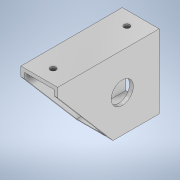
# Autodesk Inventor part: SU22_SQP_20_40_EU_sn
Saved by Autodesk Inventor 2022 (Build 260153000, 153)
## iProperties
Created: 2022-06-28
Part Number: SU22_SQP_20_40_EU_sn
Material: アルミニウム 6061-AHC
Document SubType Name: Modeling
Designer: 中島 青蔵
Density: 2.7 g/cm^3
Appearance: アルミニウム - ダーク
Author: 中島 青蔵
Autodesk Inventor part; units mm, degrees
ref_plane "YZ Plane" through (0, 0, 0) normal (1, 0, 0) x (0, 1, 0)
ref_plane "XZ Plane" through (0, 0, 0) normal (0, 1, 0) x (-1, 0, 0)
ref_plane "XY Plane" through (0, 0, 0) normal (0, 0, 1) x (1, 0, 0)
sketch "スケッチ1" plane through (0, 0, 0) normal (0, 0, 1) x (1, 0, 0)
  line L0 (0, 0) -> (20, 0)
  line L1 (20, 0) -> (20, 40)
  line L2 (20, 40) -> (0, 40)
  line L3 (0, 40) -> (0, 0)
  line L4 (2, 2) -> (18, 2)
  line L5 (18, 2) -> (18, 38)
  line L6 (18, 38) -> (2, 38)
  line L7 (2, 38) -> (2, 2)
  dimension "d0" = 20
  dimension "d1" = 40
  dimension "d2" = 2
  constraints: 16 end point, 3 other
  measures "d0" distance of L2.end L1.end
  measures "d1" distance of L1.end L0.end
  measures "d2" distance between parallel lines of L3 L7
extrude "押し出し1" add sketch "スケッチ1" along normal blind 55
sketch "スケッチ2" plane through (20, 0, 0) normal (1, 0, 0) x (0, 0, -1)
  line L0 (0, 0) -> (0, 40) projected
  point P0 (-20, 20)
  dimension "d5" = 20
  measures "d5" distance from line of L0 point (-20, 20)
hole "穴1" at (20, 20, 20) direction (-1, 0, 0) diameter 12 depth 2
sketch "スケッチ3" plane through (0, 0, 0) normal (-1, 0, 0) x (0, 0, 1)
  line L0 (0, 40) -> (0, 0) projected
  line L1 (0, 40) -> (55, 40) projected
  point P0 (20, 20)
  point P1 (20, 11)
  point P2 (20, 29)
  dimension "d13" = 20
  dimension "d14" = 20
  dimension "d15" = 9
  dimension "d16" = 9
  constraints: 2 vertical alignment
  measures "d13" distance from line of L0 point (20, 20)
  measures "d14" distance from line of L1 point (20, 20)
  measures "d15" distance of point (20, 20) point (20, 11)
  measures "d16" distance of point (20, 20) point (20, 29)
hole "穴2" at (0, 20, 20) direction (1, 0, 0) diameter 12 depth 2
hole "穴3" at (0, 11, 20) at (0, 29, 20) direction (1, 0, 0) diameter 3.1 depth 2
sketch "スケッチ4" plane through (0, 40, 0) normal (0, 1, 0) x (1, 0, 0)
  line L0 (20, 0) -> (0, 0) projected
  point P0 (10, -7.5)
  point P1 (10, -47.5)
  dimension "d31" = 7.5
  dimension "d32" = 47.5
  measures "d31" distance from line of L0 point (10, -7.5)
  measures "d32" distance from line of L0 point (10, -47.5)
hole "穴4" at (10, 40, 7.5) at (10, 40, 47.5) direction (0, -1, 0) diameter 3.1 depth 2
sketch "スケッチ5" plane through (0, 0, 0) normal (-1, 0, 0) x (0, 0, 1)
  line L0 (0, 0) -> (55, 0) projected
  line L1 (25, 0) -> (55, 35)
  line L2 (55, 2) -> (55, 38) projected
  line L3 (55, 40) -> (55, 0) projected
  dimension "d40" = 30
  dimension "d41" = 35
  constraints: 2 end point, 2 point on line
  measures "d40" distance from line of L3 L1.start
  measures "d41" distance from line of L0 L1.end
extrude "押し出し2" cut sketch "スケッチ5" against normal blind 55
equation "\"d16\" = d15"
